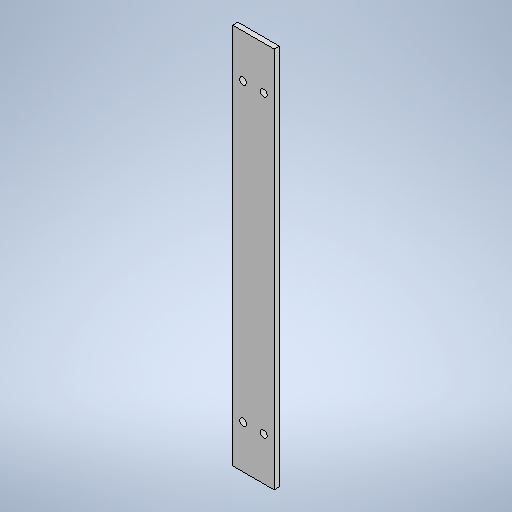
# Autodesk Inventor part: 213
Saved by Autodesk Inventor 2025 (Build 290162010, 162A)
## iProperties
Created: 2024-06-11
Part Number: 213
Material: Generic
Document SubType Name: Modeling
Designer: Fabri
Density: 1 g/cm^3
Appearance: Default
Author: Fabri
Autodesk Inventor part; units mm, degrees
ref_plane "YZ Plane" through (0, 0, 0) normal (1, 0, 0) x (0, 1, 0)
ref_plane "XZ Plane" through (0, 0, 0) normal (0, 1, 0) x (-1, 0, 0)
ref_plane "XY Plane" through (0, 0, 0) normal (0, 0, 1) x (1, 0, 0)
sketch "Sketch1" plane through (0, 0, 0) normal (0, 1, 0) x (-1, 0, 0)
  line L0 (-12, 110.5) -> (12, 110.5)
  line L1 (12, 110.5) -> (12, -110.5)
  line L2 (12, -110.5) -> (-12, -110.5)
  line L3 (-12, -110.5) -> (-12, 110.5)
  line L4 (-12, 110.5) -> (12, -110.5) construction
  line L5 (12, 110.5) -> (-12, -110.5) construction
  point P0 (0, 0)
  dimension "d0" = 24
  dimension "d1" = 221
  constraints: 12 end point, 2 midpoint, 2 parallel, 1 horizontal, 1 perpendicular
  measures "d0" distance between parallel lines of L3 L1
  measures "d1" distance between parallel lines of L2 L0
extrude "Extrusion1" add sketch "Sketch1" along normal blind 3
sketch "Sketch2" plane through (0, 3, 0) normal (0, 1, 0) x (1, 0, 0)
  line L0 (12, -110.5) -> (12, 110.5) projected
  line L1 (-12, -110.5) -> (12, -110.5) projected
  point P0 (0, 0)
  point P1 (-6, -85.5)
  point P2 (6, -85.5)
  point P3 (-6, 85.5)
  point P4 (6, 85.5)
  dimension "d4" = 12
  dimension "d5" = 6
  dimension "d6" = 171
  dimension "d7" = 25
  constraints: 2 horizontal alignment, 2 vertical alignment
  measures "d4" distance of point (6, -85.5) point (-6, -85.5)
  measures "d5" distance from line of L0 point (6, -85.5)
  measures "d6" distance of point (6, 85.5) point (6, -85.5)
  measures "d7" distance from line of L1 point (6, -85.5)
hole "Hole1" at (-6, 3, 85.5) at (6, 3, 85.5) at (-6, 3, -85.5) at (6, 3, -85.5) direction (0, -1, 0) diameter 4 depth 3
body "Solid1"
